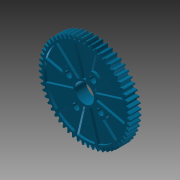
# Autodesk Inventor part: 12-0056_Gear
Saved by Autodesk Inventor 2015 SP1 (Build 190203100, 203)
## iProperties
Category: Gear Kit
Company: Autodesk Inc.
Created: 2014-11-29
Part Number: 12-0056_Gear
Material: Polystyrene, High Impact
Document SubType Name: Modeling
Designer: Matrix
Density: 1.022 g/cm^3
Appearance: Sky Blue Dark
Catalog Web Link: http://matrixrobotics.com/
Vendor: Matrix
Author: Autodesk Inc.
Autodesk Inventor part; units mm, degrees
ref_plane "YZ Plane" through (0, 0, 0) normal (1, 0, 0) x (0, 1, 0)
ref_plane "XZ Plane" through (0, 0, 0) normal (0, 1, 0) x (-1, 0, 0)
sketch "Sketch1" plane through (0, 0, 0) normal (0, 1, 0) x (-1, 0, 0)
  arc A0 (6.7425, 25.8863) -> (6.1348, 26.037) centre (0, 0) ccw
  arc A1 (5.9812, 26.2168) -> (6.1348, 26.037) centre (6.1806, 26.2317) ccw
  line L0 (5.9812, 26.2168) -> (5.8978, 27.33)
  line L1 (5.8978, 27.33) -> (5.7599, 28.1729)
  arc A2 (5.7599, 28.1729) -> (5.5196, 28.4193) centre (5.4639, 28.1245) ccw
  line L2 (5.5196, 28.4193) -> (5.2446, 28.4713)
  arc A3 (5.2446, 28.4713) -> (4.931, 28.3298) centre (5.1889, 28.1765) ccw
  line L3 (4.931, 28.3298) -> (4.4947, 27.5955)
  line L4 (4.4947, 27.5955) -> (4.0103, 26.5897)
  arc A4 (3.8017, 26.4785) -> (4.0103, 26.5897) centre (3.8301, 26.6764) ccw
  arc A5 (3.8017, 26.4785) -> (3.181, 26.5602) centre (0, 0) ccw
  arc A6 (3.0082, 26.7216) -> (3.181, 26.5602) centre (3.2047, 26.7588) ccw
  line L5 (3.0082, 26.7216) -> (2.8007, 27.8185)
  line L6 (2.8007, 27.8185) -> (2.5694, 28.6407)
  arc A7 (2.5694, 28.6407) -> (2.303, 28.8586) centre (2.2806, 28.5594) ccw
  line L7 (2.303, 28.8586) -> (2.0239, 28.8795)
  arc A8 (2.0239, 28.8795) -> (1.728, 28.7037) centre (2.0015, 28.5803) ccw
  line L8 (1.728, 28.7037) -> (1.3767, 27.9252)
  line L9 (1.3767, 27.9252) -> (1.008, 26.8715)
  arc A9 (0.8132, 26.7376) -> (1.008, 26.8715) centre (0.8192, 26.9375) ccw
  arc A10 (0.8132, 26.7376) -> (0.1872, 26.7493) centre (0, 0) ccw
  arc A11 (-0.0026, 26.8904) -> (0.1872, 26.7493) centre (0.1886, 26.9493) ccw
  line L10 (-0.0026, 26.8904) -> (-0.3316, 27.9572)
  line L11 (-0.3316, 27.9572) -> (-0.6535, 28.7483)
  arc A12 (-0.6535, 28.7483) -> (-0.9426, 28.935) centre (-0.9314, 28.6352) ccw
  line L12 (-0.9426, 28.935) -> (-1.2223, 28.9245)
  arc A13 (-1.2223, 28.9245) -> (-1.4966, 28.7167) centre (-1.2111, 28.6247) ccw
  line L13 (-1.7586, 27.9038) -> (-1.4966, 28.7167)
  line L14 (-1.7586, 27.9038) -> (-2.007, 26.8154)
  arc A14 (-2.1856, 26.6606) -> (-2.007, 26.8154) centre (-2.202, 26.8599) ccw
  arc A15 (-2.1856, 26.6606) -> (-2.809, 26.6021) centre (0, 0) ccw
  arc A16 (-3.0133, 26.721) -> (-2.809, 26.6021) centre (-2.83, 26.801) ccw
  line L15 (-3.0133, 26.721) -> (-3.4597, 27.7442)
  line L16 (-3.4597, 27.7442) -> (-3.8682, 28.4943)
  arc A17 (-3.8682, 28.4943) -> (-4.1764, 28.6475) centre (-4.1317, 28.3509) ccw
  line L17 (-4.1764, 28.6475) -> (-4.4531, 28.6058)
  arc A18 (-4.4531, 28.6058) -> (-4.7025, 28.3686) centre (-4.4084, 28.3091) ccw
  line L18 (-4.7025, 28.3686) -> (-4.8717, 27.5314)
  line L19 (-4.8717, 27.5314) -> (-4.9967, 26.4221)
  arc A19 (-5.1569, 26.2482) -> (-4.9967, 26.4221) centre (-5.1955, 26.4445) ccw
  arc A20 (-5.1569, 26.2482) -> (-5.7698, 26.1203) centre (0, 0) ccw
  arc A21 (-5.9862, 26.2156) -> (-5.7698, 26.1203) centre (-5.813, 26.3156) ccw
  line L20 (-5.9862, 26.2156) -> (-6.5444, 27.1824)
  line L21 (-6.5444, 27.1824) -> (-7.0343, 27.8821)
  arc A22 (-7.0343, 27.8821) -> (-7.3576, 27.9998) centre (-7.28, 27.71) ccw
  line L22 (-7.3576, 27.9998) -> (-7.628, 27.9273)
  arc A23 (-7.628, 27.9273) -> (-7.8492, 27.6637) centre (-7.5503, 27.6376) ccw
  line L23 (-7.8492, 27.6637) -> (-7.9236, 26.8128)
  line L24 (-7.9236, 26.8128) -> (-7.9236, 25.6965)
  arc A24 (-8.0633, 25.5058) -> (-7.9236, 25.6965) centre (-8.1236, 25.6965) ccw
  arc A25 (-8.0633, 25.5058) -> (-8.6581, 25.3101) centre (0, 0) ccw
  arc A26 (-8.8837, 25.3805) -> (-8.6581, 25.3101) centre (-8.7228, 25.4993) ccw
  line L25 (-8.8837, 25.3805) -> (-9.5467, 26.2788)
  line L26 (-9.5467, 26.2788) -> (-10.1118, 26.9192)
  arc A27 (-10.1118, 26.9192) -> (-10.4464, 26.9999) centre (-10.3368, 26.7207) ccw
  line L27 (-10.4464, 26.9999) -> (-10.7069, 26.8977)
  arc A28 (-10.7069, 26.8977) -> (-10.8972, 26.6109) centre (-10.5973, 26.6184) ccw
  line L28 (-10.8972, 26.6109) -> (-10.8759, 25.7571)
  line L29 (-10.8759, 25.7571) -> (-10.7509, 24.6477)
  arc A29 (-10.8684, 24.4426) -> (-10.7509, 24.6477) centre (-10.9496, 24.6253) ccw
  arc A30 (-10.8684, 24.4426) -> (-11.4375, 24.1815) centre (0, 0) ccw
  arc A31 (-11.6696, 24.2263) -> (-11.4375, 24.1815) centre (-11.523, 24.3623) ccw
  line L30 (-11.6696, 24.2263) -> (-12.4289, 25.0446)
  line L31 (-12.4289, 25.0446) -> (-13.0622, 25.6177)
  arc A32 (-13.0622, 25.6177) -> (-13.4037, 25.6605) centre (-13.2635, 25.3953) ccw
  line L32 (-13.4037, 25.6605) -> (-13.6511, 25.5298)
  arc A33 (-13.6511, 25.5298) -> (-13.8082, 25.2235) centre (-13.511, 25.2645) ccw
  line L33 (-13.8082, 25.2235) -> (-13.6914, 24.3774)
  line L34 (-13.6914, 24.3774) -> (-13.443, 23.289)
  arc A34 (-13.5368, 23.072) -> (-13.443, 23.289) centre (-13.638, 23.2445) ccw
  arc A35 (-13.5368, 23.072) -> (-14.073, 22.7489) centre (0, 0) ccw
  arc A36 (-14.3087, 22.7674) -> (-14.073, 22.7489) centre (-14.1783, 22.919) ccw
  line L35 (-14.3087, 22.7674) -> (-15.1549, 23.4956)
  line L36 (-15.1549, 23.4956) -> (-15.8484, 23.9942)
  arc A37 (-15.8484, 23.9942) -> (-16.1925, 23.9984) centre (-16.0235, 23.7506) ccw
  line L37 (-16.1925, 23.9984) -> (-16.4237, 23.8408)
  arc A38 (-16.4237, 23.8408) -> (-16.5455, 23.5189) centre (-16.2547, 23.5929) ccw
  line L38 (-16.5455, 23.5189) -> (-16.3347, 22.6912)
  line L39 (-16.3347, 22.6912) -> (-15.966, 21.6375)
  arc A39 (-16.0349, 21.4113) -> (-15.966, 21.6375) centre (-16.1548, 21.5714) ccw
  arc A40 (-16.0349, 21.4113) -> (-16.5316, 21.0302) centre (0, 0) ccw
  arc A41 (-16.7679, 21.0222) -> (-16.5316, 21.0302) centre (-16.6552, 21.1874) ccw
  line L40 (-16.7679, 21.0222) -> (-17.6903, 21.651)
  line L41 (-17.6903, 21.651) -> (-18.4352, 22.0688)
  arc A42 (-18.4352, 22.0688) -> (-18.7777, 22.0346) centre (-18.582, 21.8072) ccw
  line L42 (-18.7777, 22.0346) -> (-18.9898, 21.852)
  arc A43 (-18.9898, 21.852) -> (-19.0747, 21.5185) centre (-18.7941, 21.6246) ccw
  line L43 (-19.0747, 21.5185) -> (-18.7726, 20.7196)
  line L44 (-18.7726, 20.7196) -> (-18.2882, 19.7138)
  arc A44 (-18.3314, 19.4814) -> (-18.2882, 19.7138) centre (-18.4684, 19.627) ccw
  arc A45 (-18.3314, 19.4814) -> (-18.7823, 19.047) centre (0, 0) ccw
  arc A46 (-19.0162, 19.0126) -> (-18.7823, 19.047) centre (-18.9227, 19.1894) ccw
  line L45 (-19.0162, 19.0126) -> (-20.0032, 19.5342)
  line L46 (-20.0032, 19.5342) -> (-20.7902, 19.866)
  arc A47 (-20.7902, 19.866) -> (-21.1267, 19.7936) centre (-20.9068, 19.5895) ccw
  line L47 (-21.1267, 19.7936) -> (-21.317, 19.5884)
  arc A48 (-21.317, 19.5884) -> (-21.3641, 19.2475) centre (-21.0971, 19.3844) ccw
  line L48 (-21.3641, 19.2475) -> (-20.9744, 18.4875)
  line L49 (-20.9744, 18.4875) -> (-20.3805, 17.5422)
  arc A49 (-20.3973, 17.3064) -> (-20.3805, 17.5422) centre (-20.5498, 17.4358) ccw
  arc A50 (-20.3973, 17.3064) -> (-20.7968, 16.8243) centre (0, 0) ccw
  arc A51 (-21.0253, 16.7639) -> (-20.7968, 16.8243) centre (-20.9523, 16.9501) ccw
  line L50 (-21.0253, 16.7639) -> (-22.0645, 17.1717)
  line L51 (-22.8838, 17.4133) -> (-22.0645, 17.1717)
  arc A52 (-22.8838, 17.4133) -> (-23.21, 17.3037) centre (-22.9686, 17.1255) ccw
  line L52 (-23.21, 17.3037) -> (-23.3762, 17.0785)
  arc A53 (-23.3762, 17.0785) -> (-23.3848, 16.7345) centre (-23.1348, 16.9004) ccw
  line L53 (-23.3848, 16.7345) -> (-22.9125, 16.0228)
  line L54 (-22.9125, 16.0228) -> (-22.2164, 15.15)
  arc A54 (-22.2068, 14.9138) -> (-22.2164, 15.15) centre (-22.3728, 15.0253) ccw
  arc A55 (-22.2068, 14.9138) -> (-22.5497, 14.39) centre (0, 0) ccw
  arc A56 (-22.7701, 14.3044) -> (-22.5497, 14.39) centre (-22.7183, 14.4976) ccw
  line L55 (-22.7701, 14.3044) -> (-23.8484, 14.5933)
  line L56 (-23.8484, 14.5933) -> (-24.6896, 14.7416)
  arc A57 (-24.6896, 14.7416) -> (-25.0015, 14.5962) centre (-24.7417, 14.4462) ccw
  line L57 (-25.0015, 14.5962) -> (-25.1414, 14.3538)
  arc A58 (-25.1414, 14.3538) -> (-25.1114, 14.011) centre (-24.8816, 14.2038) ccw
  line L58 (-25.1114, 14.011) -> (-24.5624, 13.3567)
  line L59 (-24.5624, 13.3567) -> (-23.773, 12.5673)
  arc A59 (-23.737, 12.3337) -> (-23.773, 12.5673) centre (-23.9144, 12.4259) ccw
  arc A60 (-23.737, 12.3337) -> (-24.0191, 11.7747) centre (0, 0) ccw
  arc A61 (-24.2285, 11.665) -> (-24.0191, 11.7747) centre (-24.1987, 11.8628) ccw
  line L60 (-24.2285, 11.665) -> (-25.3324, 11.8314)
  line L61 (-25.3324, 11.8314) -> (-26.1849, 11.8846)
  arc A62 (-26.1849, 11.8846) -> (-26.4785, 11.7051) centre (-26.2035, 11.5852) ccw
  line L62 (-26.4785, 11.7051) -> (-26.5904, 11.4486)
  arc A63 (-26.5904, 11.4486) -> (-26.5222, 11.1113) centre (-26.3155, 11.3286) ccw
  line L63 (-26.5222, 11.1113) -> (-25.9034, 10.5226)
  line L64 (-25.9034, 10.5226) -> (-25.0306, 9.8265)
  arc A64 (-24.9686, 9.5984) -> (-25.0306, 9.8265) centre (-25.1553, 9.6702) ccw
  arc A65 (-24.9686, 9.5984) -> (-25.1864, 9.0114) centre (0, 0) ccw
  arc A66 (-25.3822, 8.8789) -> (-25.1864, 9.0114) centre (-25.3748, 9.0788) ccw
  line L65 (-25.3822, 8.8789) -> (-26.4978, 8.9207)
  line L66 (-26.4978, 8.9207) -> (-27.3509, 8.8781)
  arc A67 (-27.3509, 8.8781) -> (-27.6226, 8.6669) centre (-27.3359, 8.5785) ccw
  line L67 (-27.7051, 8.3994) -> (-27.6226, 8.6669)
  arc A68 (-27.7051, 8.3994) -> (-27.5995, 8.0719) centre (-27.4184, 8.311) ccw
  line L68 (-27.5995, 8.0719) -> (-26.9187, 7.5562)
  line L69 (-26.9187, 7.5562) -> (-25.9735, 6.9622)
  arc A69 (-25.8863, 6.7425) -> (-25.9735, 6.9622) centre (-26.0799, 6.7929) ccw
  arc A70 (-25.8863, 6.7425) -> (-26.037, 6.1348) centre (0, 0) ccw
  arc A71 (-26.2168, 5.9812) -> (-26.037, 6.1348) centre (-26.2317, 6.1806) ccw
  line L70 (-26.2168, 5.9812) -> (-27.33, 5.8978)
  line L71 (-27.33, 5.8978) -> (-28.1729, 5.7599)
  arc A72 (-28.1729, 5.7599) -> (-28.4193, 5.5196) centre (-28.1245, 5.4639) ccw
  line L72 (-28.4193, 5.5196) -> (-28.4713, 5.2446)
  arc A73 (-28.4713, 5.2446) -> (-28.3298, 4.931) centre (-28.1765, 5.1889) ccw
  line L73 (-28.3298, 4.931) -> (-27.5955, 4.4947)
  line L74 (-27.5955, 4.4947) -> (-26.5897, 4.0103)
  arc A74 (-26.4785, 3.8017) -> (-26.5897, 4.0103) centre (-26.6764, 3.8301) ccw
  arc A75 (-26.4785, 3.8017) -> (-26.5602, 3.181) centre (0, 0) ccw
  arc A76 (-26.7216, 3.0082) -> (-26.5602, 3.181) centre (-26.7588, 3.2047) ccw
  line L75 (-26.7216, 3.0082) -> (-27.8185, 2.8007)
  line L76 (-27.8185, 2.8007) -> (-28.6407, 2.5694)
  arc A77 (-28.6407, 2.5694) -> (-28.8586, 2.303) centre (-28.5594, 2.2806) ccw
  line L77 (-28.8586, 2.303) -> (-28.8795, 2.0239)
  arc A78 (-28.8795, 2.0239) -> (-28.7037, 1.728) centre (-28.5803, 2.0015) ccw
  line L78 (-28.7037, 1.728) -> (-27.9252, 1.3767)
  line L79 (-27.9252, 1.3767) -> (-26.8715, 1.008)
  arc A79 (-26.7376, 0.8132) -> (-26.8715, 1.008) centre (-26.9375, 0.8192) ccw
  arc A80 (-26.7376, 0.8132) -> (-26.7493, 0.1872) centre (0, 0) ccw
  arc A81 (-26.8904, -0.0026) -> (-26.7493, 0.1872) centre (-26.9493, 0.1886) ccw
  line L80 (-26.8904, -0.0026) -> (-27.9572, -0.3316)
  line L81 (-27.9572, -0.3316) -> (-28.7483, -0.6535)
  arc A82 (-28.7483, -0.6535) -> (-28.935, -0.9426) centre (-28.6352, -0.9314) ccw
  line L82 (-28.935, -0.9426) -> (-28.9245, -1.2223)
  arc A83 (-28.9245, -1.2223) -> (-28.7167, -1.4966) centre (-28.6247, -1.2111) ccw
  line L83 (-27.9038, -1.7586) -> (-28.7167, -1.4966)
  line L84 (-27.9038, -1.7586) -> (-26.8154, -2.007)
  arc A84 (-26.6606, -2.1856) -> (-26.8154, -2.007) centre (-26.8599, -2.202) ccw
  arc A85 (-26.6606, -2.1856) -> (-26.6021, -2.809) centre (0, 0) ccw
  arc A86 (-26.721, -3.0133) -> (-26.6021, -2.809) centre (-26.801, -2.83) ccw
  line L85 (-26.721, -3.0133) -> (-27.7442, -3.4597)
  line L86 (-27.7442, -3.4597) -> (-28.4943, -3.8682)
  arc A87 (-28.4943, -3.8682) -> (-28.6475, -4.1764) centre (-28.3509, -4.1317) ccw
  line L87 (-28.6475, -4.1764) -> (-28.6058, -4.4531)
  arc A88 (-28.6058, -4.4531) -> (-28.3686, -4.7025) centre (-28.3091, -4.4084) ccw
  line L88 (-28.3686, -4.7025) -> (-27.5314, -4.8717)
  line L89 (-27.5314, -4.8717) -> (-26.4221, -4.9967)
  arc A89 (-26.2482, -5.1569) -> (-26.4221, -4.9967) centre (-26.4445, -5.1955) ccw
  arc A90 (-26.2482, -5.1569) -> (-26.1203, -5.7698) centre (0, 0) ccw
  arc A91 (-26.2156, -5.9862) -> (-26.1203, -5.7698) centre (-26.3156, -5.813) ccw
  line L90 (-26.2156, -5.9862) -> (-27.1824, -6.5444)
  line L91 (-27.1824, -6.5444) -> (-27.8821, -7.0343)
  arc A92 (-27.8821, -7.0343) -> (-27.9998, -7.3576) centre (-27.71, -7.28) ccw
  line L92 (-27.9998, -7.3576) -> (-27.9273, -7.628)
  arc A93 (-27.9273, -7.628) -> (-27.6637, -7.8492) centre (-27.6376, -7.5503) ccw
  line L93 (-27.6637, -7.8492) -> (-26.8128, -7.9236)
  line L94 (-26.8128, -7.9236) -> (-25.6965, -7.9236)
  arc A94 (-25.5058, -8.0633) -> (-25.6965, -7.9236) centre (-25.6965, -8.1236) ccw
  arc A95 (-25.5058, -8.0633) -> (-25.3101, -8.6581) centre (0, 0) ccw
  arc A96 (-25.3805, -8.8837) -> (-25.3101, -8.6581) centre (-25.4993, -8.7228) ccw
  line L95 (-25.3805, -8.8837) -> (-26.2788, -9.5467)
  line L96 (-26.2788, -9.5467) -> (-26.9192, -10.1118)
  arc A97 (-26.9192, -10.1118) -> (-26.9999, -10.4464) centre (-26.7207, -10.3368) ccw
  line L97 (-26.9999, -10.4464) -> (-26.8977, -10.7069)
  arc A98 (-26.8977, -10.7069) -> (-26.6109, -10.8972) centre (-26.6184, -10.5973) ccw
  line L98 (-26.6109, -10.8972) -> (-25.7571, -10.8759)
  line L99 (-25.7571, -10.8759) -> (-24.6477, -10.7509)
  arc A99 (-24.4426, -10.8684) -> (-24.6477, -10.7509) centre (-24.6253, -10.9496) ccw
  arc A100 (-24.4426, -10.8684) -> (-24.1815, -11.4375) centre (0, 0) ccw
  arc A101 (-24.2263, -11.6696) -> (-24.1815, -11.4375) centre (-24.3623, -11.523) ccw
  line L100 (-24.2263, -11.6696) -> (-25.0446, -12.4289)
  line L101 (-25.0446, -12.4289) -> (-25.6177, -13.0622)
  arc A102 (-25.6177, -13.0622) -> (-25.6605, -13.4037) centre (-25.3953, -13.2635) ccw
  line L102 (-25.6605, -13.4037) -> (-25.5298, -13.6511)
  arc A103 (-25.5298, -13.6511) -> (-25.2235, -13.8082) centre (-25.2645, -13.511) ccw
  line L103 (-25.2235, -13.8082) -> (-24.3774, -13.6914)
  line L104 (-24.3774, -13.6914) -> (-23.289, -13.443)
  arc A104 (-23.072, -13.5368) -> (-23.289, -13.443) centre (-23.2445, -13.638) ccw
  arc A105 (-23.072, -13.5368) -> (-22.7489, -14.073) centre (0, 0) ccw
  arc A106 (-22.7674, -14.3087) -> (-22.7489, -14.073) centre (-22.919, -14.1783) ccw
  line L105 (-22.7674, -14.3087) -> (-23.4956, -15.1549)
  line L106 (-23.4956, -15.1549) -> (-23.9942, -15.8484)
  arc A107 (-23.9942, -15.8484) -> (-23.9984, -16.1925) centre (-23.7506, -16.0235) ccw
  line L107 (-23.9984, -16.1925) -> (-23.8408, -16.4237)
  arc A108 (-23.8408, -16.4237) -> (-23.5189, -16.5455) centre (-23.5929, -16.2547) ccw
  line L108 (-23.5189, -16.5455) -> (-22.6912, -16.3347)
  line L109 (-22.6912, -16.3347) -> (-21.6375, -15.966)
  arc A109 (-21.4113, -16.0349) -> (-21.6375, -15.966) centre (-21.5714, -16.1548) ccw
  arc A110 (-21.4113, -16.0349) -> (-21.0302, -16.5316) centre (0, 0) ccw
  arc A111 (-21.0222, -16.7679) -> (-21.0302, -16.5316) centre (-21.1874, -16.6552) ccw
  line L110 (-21.0222, -16.7679) -> (-21.651, -17.6903)
  line L111 (-21.651, -17.6903) -> (-22.0688, -18.4352)
  arc A112 (-22.0688, -18.4352) -> (-22.0346, -18.7777) centre (-21.8072, -18.582) ccw
  line L112 (-22.0346, -18.7777) -> (-21.852, -18.9898)
  arc A113 (-21.852, -18.9898) -> (-21.5185, -19.0747) centre (-21.6246, -18.7941) ccw
  line L113 (-21.5185, -19.0747) -> (-20.7196, -18.7726)
  line L114 (-20.7196, -18.7726) -> (-19.7138, -18.2882)
  arc A114 (-19.4814, -18.3314) -> (-19.7138, -18.2882) centre (-19.627, -18.4684) ccw
  arc A115 (-19.4814, -18.3314) -> (-19.047, -18.7823) centre (0, 0) ccw
  arc A116 (-19.0126, -19.0162) -> (-19.047, -18.7823) centre (-19.1894, -18.9227) ccw
  line L115 (-19.0126, -19.0162) -> (-19.5342, -20.0032)
  line L116 (-19.5342, -20.0032) -> (-19.866, -20.7902)
  arc A117 (-19.866, -20.7902) -> (-19.7936, -21.1267) centre (-19.5895, -20.9068) ccw
  line L117 (-19.7936, -21.1267) -> (-19.5884, -21.317)
  arc A118 (-19.5884, -21.317) -> (-19.2475, -21.3641) centre (-19.3844, -21.0971) ccw
  line L118 (-19.2475, -21.3641) -> (-18.4875, -20.9744)
  line L119 (-18.4875, -20.9744) -> (-17.5422, -20.3805)
  arc A119 (-17.3064, -20.3973) -> (-17.5422, -20.3805) centre (-17.4358, -20.5498) ccw
  arc A120 (-17.3064, -20.3973) -> (-16.8243, -20.7968) centre (0, 0) ccw
  arc A121 (-16.7639, -21.0253) -> (-16.8243, -20.7968) centre (-16.9501, -20.9523) ccw
  line L120 (-16.7639, -21.0253) -> (-17.1717, -22.0645)
  line L121 (-17.4133, -22.8838) -> (-17.1717, -22.0645)
  arc A122 (-17.4133, -22.8838) -> (-17.3037, -23.21) centre (-17.1255, -22.9686) ccw
  line L122 (-17.3037, -23.21) -> (-17.0785, -23.3762)
  arc A123 (-17.0785, -23.3762) -> (-16.7345, -23.3848) centre (-16.9004, -23.1348) ccw
  line L123 (-16.7345, -23.3848) -> (-16.0228, -22.9125)
  line L124 (-16.0228, -22.9125) -> (-15.15, -22.2164)
  arc A124 (-14.9138, -22.2068) -> (-15.15, -22.2164) centre (-15.0253, -22.3728) ccw
  arc A125 (-14.9138, -22.2068) -> (-14.39, -22.5497) centre (0, 0) ccw
  arc A126 (-14.3044, -22.7701) -> (-14.39, -22.5497) centre (-14.4976, -22.7183) ccw
  line L125 (-14.3044, -22.7701) -> (-14.5933, -23.8484)
  line L126 (-14.5933, -23.8484) -> (-14.7416, -24.6896)
  arc A127 (-14.7416, -24.6896) -> (-14.5962, -25.0015) centre (-14.4462, -24.7417) ccw
  line L127 (-14.5962, -25.0015) -> (-14.3538, -25.1414)
  arc A128 (-14.3538, -25.1414) -> (-14.011, -25.1114) centre (-14.2038, -24.8816) ccw
  line L128 (-14.011, -25.1114) -> (-13.3567, -24.5624)
  line L129 (-13.3567, -24.5624) -> (-12.5673, -23.773)
  arc A129 (-12.3337, -23.737) -> (-12.5673, -23.773) centre (-12.4259, -23.9144) ccw
  arc A130 (-12.3337, -23.737) -> (-11.7747, -24.0191) centre (0, 0) ccw
  arc A131 (-11.665, -24.2285) -> (-11.7747, -24.0191) centre (-11.8628, -24.1987) ccw
  line L130 (-11.665, -24.2285) -> (-11.8314, -25.3324)
  line L131 (-11.8314, -25.3324) -> (-11.8846, -26.1849)
  arc A132 (-11.8846, -26.1849) -> (-11.7051, -26.4785) centre (-11.5852, -26.2035) ccw
  line L132 (-11.7051, -26.4785) -> (-11.4486, -26.5904)
  arc A133 (-11.4486, -26.5904) -> (-11.1113, -26.5222) centre (-11.3286, -26.3155) ccw
  line L133 (-11.1113, -26.5222) -> (-10.5226, -25.9034)
  line L134 (-10.5226, -25.9034) -> (-9.8265, -25.0306)
  arc A134 (-9.5984, -24.9686) -> (-9.8265, -25.0306) centre (-9.6702, -25.1553) ccw
  arc A135 (-9.5984, -24.9686) -> (-9.0114, -25.1864) centre (0, 0) ccw
  arc A136 (-8.8789, -25.3822) -> (-9.0114, -25.1864) centre (-9.0788, -25.3748) ccw
  line L135 (-8.8789, -25.3822) -> (-8.9207, -26.4978)
  line L136 (-8.9207, -26.4978) -> (-8.8781, -27.3509)
  arc A137 (-8.8781, -27.3509) -> (-8.6669, -27.6226) centre (-8.5785, -27.3359) ccw
  line L137 (-8.3994, -27.7051) -> (-8.6669, -27.6226)
  arc A138 (-8.3994, -27.7051) -> (-8.0719, -27.5995) centre (-8.311, -27.4184) ccw
  line L138 (-8.0719, -27.5995) -> (-7.5562, -26.9187)
  line L139 (-7.5562, -26.9187) -> (-6.9622, -25.9735)
  arc A139 (-6.7425, -25.8863) -> (-6.9622, -25.9735) centre (-6.7929, -26.0799) ccw
  arc A140 (-6.7425, -25.8863) -> (-6.1348, -26.037) centre (0, 0) ccw
  arc A141 (-5.9812, -26.2168) -> (-6.1348, -26.037) centre (-6.1806, -26.2317) ccw
  line L140 (-5.9812, -26.2168) -> (-5.8978, -27.33)
  line L141 (-5.8978, -27.33) -> (-5.7599, -28.1729)
  arc A142 (-5.7599, -28.1729) -> (-5.5196, -28.4193) centre (-5.4639, -28.1245) ccw
  line L142 (-5.5196, -28.4193) -> (-5.2446, -28.4713)
  arc A143 (-5.2446, -28.4713) -> (-4.931, -28.3298) centre (-5.1889, -28.1765) ccw
  line L143 (-4.931, -28.3298) -> (-4.4947, -27.5955)
  line L144 (-4.4947, -27.5955) -> (-4.0103, -26.5897)
  arc A144 (-3.8017, -26.4785) -> (-4.0103, -26.5897) centre (-3.8301, -26.6764) ccw
  arc A145 (-3.8017, -26.4785) -> (-3.181, -26.5602) centre (0, 0) ccw
  arc A146 (-3.0082, -26.7216) -> (-3.181, -26.5602) centre (-3.2047, -26.7588) ccw
  line L145 (-3.0082, -26.7216) -> (-2.8007, -27.8185)
  line L146 (-2.8007, -27.8185) -> (-2.5694, -28.6407)
  arc A147 (-2.5694, -28.6407) -> (-2.303, -28.8586) centre (-2.2806, -28.5594) ccw
  line L147 (-2.303, -28.8586) -> (-2.0239, -28.8795)
  arc A148 (-2.0239, -28.8795) -> (-1.728, -28.7037) centre (-2.0015, -28.5803) ccw
  line L148 (-1.728, -28.7037) -> (-1.3767, -27.9252)
  line L149 (-1.3767, -27.9252) -> (-1.008, -26.8715)
  arc A149 (-0.8132, -26.7376) -> (-1.008, -26.8715) centre (-0.8192, -26.9375) ccw
  arc A150 (-0.8132, -26.7376) -> (-0.1872, -26.7493) centre (0, 0) ccw
  arc A151 (0.0026, -26.8904) -> (-0.1872, -26.7493) centre (-0.1886, -26.9493) ccw
  line L150 (0.0026, -26.8904) -> (0.3316, -27.9572)
  line L151 (0.3316, -27.9572) -> (0.6535, -28.7483)
  arc A152 (0.6535, -28.7483) -> (0.9426, -28.935) centre (0.9314, -28.6352) ccw
  line L152 (0.9426, -28.935) -> (1.2223, -28.9245)
  arc A153 (1.2223, -28.9245) -> (1.4966, -28.7167) centre (1.2111, -28.6247) ccw
  line L153 (1.7586, -27.9038) -> (1.4966, -28.7167)
  line L154 (1.7586, -27.9038) -> (2.007, -26.8154)
  arc A154 (2.1856, -26.6606) -> (2.007, -26.8154) centre (2.202, -26.8599) ccw
  arc A155 (2.1856, -26.6606) -> (2.809, -26.6021) centre (0, 0) ccw
  arc A156 (3.0133, -26.721) -> (2.809, -26.6021) centre (2.83, -26.801) ccw
  line L155 (3.0133, -26.721) -> (3.4597, -27.7442)
  line L156 (3.4597, -27.7442) -> (3.8682, -28.4943)
  arc A157 (3.8682, -28.4943) -> (4.1764, -28.6475) centre (4.1317, -28.3509) ccw
  line L157 (4.1764, -28.6475) -> (4.4531, -28.6058)
  arc A158 (4.4531, -28.6058) -> (4.7025, -28.3686) centre (4.4084, -28.3091) ccw
  line L158 (4.7025, -28.3686) -> (4.8717, -27.5314)
  line L159 (4.8717, -27.5314) -> (4.9967, -26.4221)
  arc A159 (5.1569, -26.2482) -> (4.9967, -26.4221) centre (5.1955, -26.4445) ccw
  arc A160 (5.1569, -26.2482) -> (5.7698, -26.1203) centre (0, 0) ccw
  arc A161 (5.9862, -26.2156) -> (5.7698, -26.1203) centre (5.813, -26.3156) ccw
  line L160 (5.9862, -26.2156) -> (6.5444, -27.1824)
  line L161 (6.5444, -27.1824) -> (7.0343, -27.8821)
  arc A162 (7.0343, -27.8821) -> (7.3576, -27.9998) centre (7.28, -27.71) ccw
  line L162 (7.3576, -27.9998) -> (7.628, -27.9273)
  arc A163 (7.628, -27.9273) -> (7.8492, -27.6637) centre (7.5503, -27.6376) ccw
  line L163 (7.8492, -27.6637) -> (7.9236, -26.8128)
  line L164 (7.9236, -26.8128) -> (7.9236, -25.6965)
  arc A164 (8.0633, -25.5058) -> (7.9236, -25.6965) centre (8.1236, -25.6965) ccw
  arc A165 (8.0633, -25.5058) -> (8.6581, -25.3101) centre (0, 0) ccw
  arc A166 (8.8837, -25.3805) -> (8.6581, -25.3101) centre (8.7228, -25.4993) ccw
  line L165 (8.8837, -25.3805) -> (9.5467, -26.2788)
  line L166 (9.5467, -26.2788) -> (10.1118, -26.9192)
  arc A167 (10.1118, -26.9192) -> (10.4464, -26.9999) centre (10.3368, -26.7207) ccw
  line L167 (10.4464, -26.9999) -> (10.7069, -26.8977)
  arc A168 (10.7069, -26.8977) -> (10.8972, -26.6109) centre (10.5973, -26.6184) ccw
  line L168 (10.8972, -26.6109) -> (10.8759, -25.7571)
  line L169 (10.8759, -25.7571) -> (10.7509, -24.6477)
  arc A169 (10.8684, -24.4426) -> (10.7509, -24.6477) centre (10.9496, -24.6253) ccw
  arc A170 (10.8684, -24.4426) -> (11.4375, -24.1815) centre (0, 0) ccw
  arc A171 (11.6696, -24.2263) -> (11.4375, -24.1815) centre (11.523, -24.3623) ccw
  line L170 (11.6696, -24.2263) -> (12.4289, -25.0446)
  line L171 (12.4289, -25.0446) -> (13.0622, -25.6177)
  arc A172 (13.0622, -25.6177) -> (13.4037, -25.6605) centre (13.2635, -25.3953) ccw
  line L172 (13.4037, -25.6605) -> (13.6511, -25.5298)
  arc A173 (13.6511, -25.5298) -> (13.8082, -25.2235) centre (13.511, -25.2645) ccw
  line L173 (13.8082, -25.2235) -> (13.6914, -24.3774)
  line L174 (13.6914, -24.3774) -> (13.443, -23.289)
  arc A174 (13.5368, -23.072) -> (13.443, -23.289) centre (13.638, -23.2445) ccw
  arc A175 (13.5368, -23.072) -> (14.073, -22.7489) centre (0, 0) ccw
  arc A176 (14.3087, -22.7674) -> (14.073, -22.7489) centre (14.1783, -22.919) ccw
  line L175 (14.3087, -22.7674) -> (15.1549, -23.4956)
  line L176 (15.1549, -23.4956) -> (15.8484, -23.9942)
  arc A177 (15.8484, -23.9942) -> (16.1925, -23.9984) centre (16.0235, -23.7506) ccw
  line L177 (16.1925, -23.9984) -> (16.4237, -23.8408)
  arc A178 (16.4237, -23.8408) -> (16.5455, -23.5189) centre (16.2547, -23.5929) ccw
  line L178 (16.5455, -23.5189) -> (16.3347, -22.6912)
  line L179 (16.3347, -22.6912) -> (15.966, -21.6375)
  arc A179 (16.0349, -21.4113) -> (15.966, -21.6375) centre (16.1548, -21.5714) ccw
  arc A180 (16.0349, -21.4113) -> (16.5316, -21.0302) centre (0, 0) ccw
  arc A181 (16.7679, -21.0222) -> (16.5316, -21.0302) centre (16.6552, -21.1874) ccw
  line L180 (16.7679, -21.0222) -> (17.6903, -21.651)
  line L181 (17.6903, -21.651) -> (18.4352, -22.0688)
  arc A182 (18.4352, -22.0688) -> (18.7777, -22.0346) centre (18.582, -21.8072) ccw
  line L182 (18.7777, -22.0346) -> (18.9898, -21.852)
  arc A183 (18.9898, -21.852) -> (19.0747, -21.5185) centre (18.7941, -21.6246) ccw
  line L183 (19.0747, -21.5185) -> (18.7726, -20.7196)
  line L184 (18.7726, -20.7196) -> (18.2882, -19.7138)
  arc A184 (18.3314, -19.4814) -> (18.2882, -19.7138) centre (18.4684, -19.627) ccw
  arc A185 (18.3314, -19.4814) -> (18.7823, -19.047) centre (0, 0) ccw
  arc A186 (19.0162, -19.0126) -> (18.7823, -19.047) centre (18.9227, -19.1894) ccw
  line L185 (19.0162, -19.0126) -> (20.0032, -19.5342)
  line L186 (20.0032, -19.5342) -> (20.7902, -19.866)
  arc A187 (20.7902, -19.866) -> (21.1267, -19.7936) centre (20.9068, -19.5895) ccw
  line L187 (21.1267, -19.7936) -> (21.317, -19.5884)
  arc A188 (21.317, -19.5884) -> (21.3641, -19.2475) centre (21.0971, -19.3844) ccw
  line L188 (21.3641, -19.2475) -> (20.9744, -18.4875)
  line L189 (20.9744, -18.4875) -> (20.3805, -17.5422)
  arc A189 (20.3973, -17.3064) -> (20.3805, -17.5422) centre (20.5498, -17.4358) ccw
  arc A190 (20.3973, -17.3064) -> (20.7968, -16.8243) centre (0, 0) ccw
  arc A191 (21.0253, -16.7639) -> (20.7968, -16.8243) centre (20.9523, -16.9501) ccw
  line L190 (21.0253, -16.7639) -> (22.0645, -17.1717)
  line L191 (22.8838, -17.4133) -> (22.0645, -17.1717)
  arc A192 (22.8838, -17.4133) -> (23.21, -17.3037) centre (22.9686, -17.1255) ccw
  line L192 (23.21, -17.3037) -> (23.3762, -17.0785)
  arc A193 (23.3762, -17.0785) -> (23.3848, -16.7345) centre (23.1348, -16.9004) ccw
  line L193 (23.3848, -16.7345) -> (22.9125, -16.0228)
  line L194 (22.9125, -16.0228) -> (22.2164, -15.15)
  arc A194 (22.2068, -14.9138) -> (22.2164, -15.15) centre (22.3728, -15.0253) ccw
  arc A195 (22.2068, -14.9138) -> (22.5497, -14.39) centre (0, 0) ccw
  arc A196 (22.7701, -14.3044) -> (22.5497, -14.39) centre (22.7183, -14.4976) ccw
  line L195 (22.7701, -14.3044) -> (23.8484, -14.5933)
  line L196 (23.8484, -14.5933) -> (24.6896, -14.7416)
  arc A197 (24.6896, -14.7416) -> (25.0015, -14.5962) centre (24.7417, -14.4462) ccw
  line L197 (25.0015, -14.5962) -> (25.1414, -14.3538)
  arc A198 (25.1414, -14.3538) -> (25.1114, -14.011) centre (24.8816, -14.2038) ccw
  line L198 (25.1114, -14.011) -> (24.5624, -13.3567)
  line L199 (24.5624, -13.3567) -> (23.773, -12.5673)
  arc A199 (23.737, -12.3337) -> (23.773, -12.5673) centre (23.9144, -12.4259) ccw
  arc A200 (23.737, -12.3337) -> (24.0191, -11.7747) centre (0, 0) ccw
  arc A201 (24.2285, -11.665) -> (24.0191, -11.7747) centre (24.1987, -11.8628) ccw
  line L200 (24.2285, -11.665) -> (25.3324, -11.8314)
  line L201 (25.3324, -11.8314) -> (26.1849, -11.8846)
  arc A202 (26.1849, -11.8846) -> (26.4785, -11.7051) centre (26.2035, -11.5852) ccw
  line L202 (26.4785, -11.7051) -> (26.5904, -11.4486)
  arc A203 (26.5904, -11.4486) -> (26.5222, -11.1113) centre (26.3155, -11.3286) ccw
  line L203 (26.5222, -11.1113) -> (25.9034, -10.5226)
  line L204 (25.9034, -10.5226) -> (25.0306, -9.8265)
  arc A204 (24.9686, -9.5984) -> (25.0306, -9.8265) centre (25.1553, -9.6702) ccw
  arc A205 (24.9686, -9.5984) -> (25.1864, -9.0114) centre (0, 0) ccw
  arc A206 (25.3822, -8.8789) -> (25.1864, -9.0114) centre (25.3748, -9.0788) ccw
  line L205 (25.3822, -8.8789) -> (26.4978, -8.9207)
  line L206 (26.4978, -8.9207) -> (27.3509, -8.8781)
  arc A207 (27.3509, -8.8781) -> (27.6226, -8.6669) centre (27.3359, -8.5785) ccw
  line L207 (27.7051, -8.3994) -> (27.6226, -8.6669)
  arc A208 (27.7051, -8.3994) -> (27.5995, -8.0719) centre (27.4184, -8.311) ccw
  line L208 (27.5995, -8.0719) -> (26.9187, -7.5562)
  line L209 (26.9187, -7.5562) -> (25.9735, -6.9622)
  arc A209 (25.8863, -6.7425) -> (25.9735, -6.9622) centre (26.0799, -6.7929) ccw
  arc A210 (25.8863, -6.7425) -> (26.037, -6.1348) centre (0, 0) ccw
  arc A211 (26.2168, -5.9812) -> (26.037, -6.1348) centre (26.2317, -6.1806) ccw
  line L210 (26.2168, -5.9812) -> (27.33, -5.8978)
  line L211 (27.33, -5.8978) -> (28.1729, -5.7599)
  arc A212 (28.1729, -5.7599) -> (28.4193, -5.5196) centre (28.1245, -5.4639) ccw
  line L212 (28.4193, -5.5196) -> (28.4713, -5.2446)
  arc A213 (28.4713, -5.2446) -> (28.3298, -4.931) centre (28.1765, -5.1889) ccw
  line L213 (28.3298, -4.931) -> (27.5955, -4.4947)
  line L214 (27.5955, -4.4947) -> (26.5897, -4.0103)
  arc A214 (26.4785, -3.8017) -> (26.5897, -4.0103) centre (26.6764, -3.8301) ccw
  arc A215 (26.4785, -3.8017) -> (26.5602, -3.181) centre (0, 0) ccw
  arc A216 (26.7216, -3.0082) -> (26.5602, -3.181) centre (26.7588, -3.2047) ccw
  line L215 (26.7216, -3.0082) -> (27.8185, -2.8007)
  line L216 (27.8185, -2.8007) -> (28.6407, -2.5694)
  arc A217 (28.6407, -2.5694) -> (28.8586, -2.303) centre (28.5594, -2.2806) ccw
  line L217 (28.8586, -2.303) -> (28.8795, -2.0239)
  arc A218 (28.8795, -2.0239) -> (28.7037, -1.728) centre (28.5803, -2.0015) ccw
  line L218 (28.7037, -1.728) -> (27.9252, -1.3767)
  line L219 (27.9252, -1.3767) -> (26.8715, -1.008)
  arc A219 (26.7376, -0.8132) -> (26.8715, -1.008) centre (26.9375, -0.8192) ccw
  arc A220 (26.7376, -0.8132) -> (26.7493, -0.1872) centre (0, 0) ccw
  arc A221 (26.8904, 0.0026) -> (26.7493, -0.1872) centre (26.9493, -0.1886) ccw
  line L220 (26.8904, 0.0026) -> (27.9572, 0.3316)
  line L221 (27.9572, 0.3316) -> (28.7483, 0.6535)
  arc A222 (28.7483, 0.6535) -> (28.935, 0.9426) centre (28.6352, 0.9314) ccw
  line L222 (28.935, 0.9426) -> (28.9245, 1.2223)
  arc A223 (28.9245, 1.2223) -> (28.7167, 1.4966) centre (28.6247, 1.2111) ccw
  line L223 (27.9038, 1.7586) -> (28.7167, 1.4966)
  line L224 (27.9038, 1.7586) -> (26.8154, 2.007)
  arc A224 (26.6606, 2.1856) -> (26.8154, 2.007) centre (26.8599, 2.202) ccw
  arc A225 (26.6606, 2.1856) -> (26.6021, 2.809) centre (0, 0) ccw
  arc A226 (26.721, 3.0133) -> (26.6021, 2.809) centre (26.801, 2.83) ccw
  line L225 (26.721, 3.0133) -> (27.7442, 3.4597)
  line L226 (27.7442, 3.4597) -> (28.4943, 3.8682)
  arc A227 (28.4943, 3.8682) -> (28.6475, 4.1764) centre (28.3509, 4.1317) ccw
  line L227 (28.6475, 4.1764) -> (28.6058, 4.4531)
  arc A228 (28.6058, 4.4531) -> (28.3686, 4.7025) centre (28.3091, 4.4084) ccw
  line L228 (28.3686, 4.7025) -> (27.5314, 4.8717)
  line L229 (27.5314, 4.8717) -> (26.4221, 4.9967)
  arc A229 (26.2482, 5.1569) -> (26.4221, 4.9967) centre (26.4445, 5.1955) ccw
  arc A230 (26.2482, 5.1569) -> (26.1203, 5.7698) centre (0, 0) ccw
  arc A231 (26.2156, 5.9862) -> (26.1203, 5.7698) centre (26.3156, 5.813) ccw
  line L230 (26.2156, 5.9862) -> (27.1824, 6.5444)
  line L231 (27.1824, 6.5444) -> (27.8821, 7.0343)
  arc A232 (27.8821, 7.0343) -> (27.9998, 7.3576) centre (27.71, 7.28) ccw
  line L232 (27.9998, 7.3576) -> (27.9273, 7.628)
  arc A233 (27.9273, 7.628) -> (27.6637, 7.8492) centre (27.6376, 7.5503) ccw
  line L233 (27.6637, 7.8492) -> (26.8128, 7.9236)
  line L234 (26.8128, 7.9236) -> (25.6965, 7.9236)
  arc A234 (25.5058, 8.0633) -> (25.6965, 7.9236) centre (25.6965, 8.1236) ccw
  arc A235 (25.5058, 8.0633) -> (25.3101, 8.6581) centre (0, 0) ccw
  arc A236 (25.3805, 8.8837) -> (25.3101, 8.6581) centre (25.4993, 8.7228) ccw
  line L235 (25.3805, 8.8837) -> (26.2788, 9.5467)
  line L236 (26.2788, 9.5467) -> (26.9192, 10.1118)
  arc A237 (26.9192, 10.1118) -> (26.9999, 10.4464) centre (26.7207, 10.3368) ccw
  line L237 (26.9999, 10.4464) -> (26.8977, 10.7069)
  arc A238 (26.8977, 10.7069) -> (26.6109, 10.8972) centre (26.6184, 10.5973) ccw
  line L238 (26.6109, 10.8972) -> (25.7571, 10.8759)
  line L239 (25.7571, 10.8759) -> (24.6477, 10.7509)
  arc A239 (24.4426, 10.8684) -> (24.6477, 10.7509) centre (24.6253, 10.9496) ccw
  arc A240 (24.4426, 10.8684) -> (24.1815, 11.4375) centre (0, 0) ccw
  arc A241 (24.2263, 11.6696) -> (24.1815, 11.4375) centre (24.3623, 11.523) ccw
  line L240 (24.2263, 11.6696) -> (25.0446, 12.4289)
  line L241 (25.0446, 12.4289) -> (25.6177, 13.0622)
  arc A242 (25.6177, 13.0622) -> (25.6605, 13.4037) centre (25.3953, 13.2635) ccw
  line L242 (25.6605, 13.4037) -> (25.5298, 13.6511)
  arc A243 (25.5298, 13.6511) -> (25.2235, 13.8082) centre (25.2645, 13.511) ccw
  line L243 (25.2235, 13.8082) -> (24.3774, 13.6914)
  line L244 (24.3774, 13.6914) -> (23.289, 13.443)
  arc A244 (23.072, 13.5368) -> (23.289, 13.443) centre (23.2445, 13.638) ccw
  arc A245 (23.072, 13.5368) -> (22.7489, 14.073) centre (0, 0) ccw
  arc A246 (22.7674, 14.3087) -> (22.7489, 14.073) centre (22.919, 14.1783) ccw
  line L245 (22.7674, 14.3087) -> (23.4956, 15.1549)
  line L246 (23.4956, 15.1549) -> (23.9942, 15.8484)
  arc A247 (23.9942, 15.8484) -> (23.9984, 16.1925) centre (23.7506, 16.0235) ccw
  line L247 (23.9984, 16.1925) -> (23.8408, 16.4237)
  arc A248 (23.8408, 16.4237) -> (23.5189, 16.5455) centre (23.5929, 16.2547) ccw
  line L248 (23.5189, 16.5455) -> (22.6912, 16.3347)
  line L249 (22.6912, 16.3347) -> (21.6375, 15.966)
  arc A249 (21.4113, 16.0349) -> (21.6375, 15.966) centre (21.5714, 16.1548) ccw
  arc A250 (21.4113, 16.0349) -> (21.0302, 16.5316) centre (0, 0) ccw
  arc A251 (21.0222, 16.7679) -> (21.0302, 16.5316) centre (21.1874, 16.6552) ccw
  line L250 (21.0222, 16.7679) -> (21.651, 17.6903)
  line L251 (21.651, 17.6903) -> (22.0688, 18.4352)
  arc A252 (22.0688, 18.4352) -> (22.0346, 18.7777) centre (21.8072, 18.582) ccw
  line L252 (22.0346, 18.7777) -> (21.852, 18.9898)
  arc A253 (21.852, 18.9898) -> (21.5185, 19.0747) centre (21.6246, 18.7941) ccw
  line L253 (21.5185, 19.0747) -> (20.7196, 18.7726)
  line L254 (20.7196, 18.7726) -> (19.7138, 18.2882)
  arc A254 (19.4814, 18.3314) -> (19.7138, 18.2882) centre (19.627, 18.4684) ccw
  arc A255 (19.4814, 18.3314) -> (19.047, 18.7823) centre (0, 0) ccw
  arc A256 (19.0126, 19.0162) -> (19.047, 18.7823) centre (19.1894, 18.9227) ccw
  line L255 (19.0126, 19.0162) -> (19.5342, 20.0032)
  line L256 (19.5342, 20.0032) -> (19.866, 20.7902)
  arc A257 (19.866, 20.7902) -> (19.7936, 21.1267) centre (19.5895, 20.9068) ccw
  line L257 (19.7936, 21.1267) -> (19.5884, 21.317)
  arc A258 (19.5884, 21.317) -> (19.2475, 21.3641) centre (19.3844, 21.0971) ccw
  line L258 (19.2475, 21.3641) -> (18.4875, 20.9744)
  line L259 (18.4875, 20.9744) -> (17.5422, 20.3805)
  arc A259 (17.3064, 20.3973) -> (17.5422, 20.3805) centre (17.4358, 20.5498) ccw
  arc A260 (17.3064, 20.3973) -> (16.8243, 20.7968) centre (0, 0) ccw
  arc A261 (16.7639, 21.0253) -> (16.8243, 20.7968) centre (16.9501, 20.9523) ccw
  line L260 (16.7639, 21.0253) -> (17.1717, 22.0645)
  line L261 (17.4133, 22.8838) -> (17.1717, 22.0645)
  arc A262 (17.4133, 22.8838) -> (17.3037, 23.21) centre (17.1255, 22.9686) ccw
  line L262 (17.3037, 23.21) -> (17.0785, 23.3762)
  arc A263 (17.0785, 23.3762) -> (16.7345, 23.3848) centre (16.9004, 23.1348) ccw
  line L263 (16.7345, 23.3848) -> (16.0228, 22.9125)
  line L264 (16.0228, 22.9125) -> (15.15, 22.2164)
  arc A264 (14.9138, 22.2068) -> (15.15, 22.2164) centre (15.0253, 22.3728) ccw
  arc A265 (14.9138, 22.2068) -> (14.39, 22.5497) centre (0, 0) ccw
  arc A266 (14.3044, 22.7701) -> (14.39, 22.5497) centre (14.4976, 22.7183) ccw
  line L265 (14.3044, 22.7701) -> (14.5933, 23.8484)
  line L266 (14.5933, 23.8484) -> (14.7416, 24.6896)
  arc A267 (14.7416, 24.6896) -> (14.5962, 25.0015) centre (14.4462, 24.7417) ccw
  line L267 (14.5962, 25.0015) -> (14.3538, 25.1414)
  arc A268 (14.3538, 25.1414) -> (14.011, 25.1114) centre (14.2038, 24.8816) ccw
  line L268 (14.011, 25.1114) -> (13.3567, 24.5624)
  line L269 (13.3567, 24.5624) -> (12.5673, 23.773)
  arc A269 (12.3337, 23.737) -> (12.5673, 23.773) centre (12.4259, 23.9144) ccw
  arc A270 (12.3337, 23.737) -> (11.7747, 24.0191) centre (0, 0) ccw
  arc A271 (11.665, 24.2285) -> (11.7747, 24.0191) centre (11.8628, 24.1987) ccw
  line L270 (11.665, 24.2285) -> (11.8314, 25.3324)
  line L271 (11.8314, 25.3324) -> (11.8846, 26.1849)
  arc A272 (11.8846, 26.1849) -> (11.7051, 26.4785) centre (11.5852, 26.2035) ccw
  line L272 (11.7051, 26.4785) -> (11.4486, 26.5904)
  arc A273 (11.4486, 26.5904) -> (11.1113, 26.5222) centre (11.3286, 26.3155) ccw
  line L273 (11.1113, 26.5222) -> (10.5226, 25.9034)
  line L274 (10.5226, 25.9034) -> (9.8265, 25.0306)
  arc A274 (9.5984, 24.9686) -> (9.8265, 25.0306) centre (9.6702, 25.1553) ccw
  arc A275 (9.5984, 24.9686) -> (9.0114, 25.1864) centre (0, 0) ccw
  arc A276 (8.8789, 25.3822) -> (9.0114, 25.1864) centre (9.0788, 25.3748) ccw
  line L275 (8.8789, 25.3822) -> (8.9207, 26.4978)
  line L276 (8.9207, 26.4978) -> (8.8781, 27.3509)
  arc A277 (8.8781, 27.3509) -> (8.6669, 27.6226) centre (8.5785, 27.3359) ccw
  line L277 (8.3994, 27.7051) -> (8.6669, 27.6226)
  arc A278 (8.3994, 27.7051) -> (8.0719, 27.5995) centre (8.311, 27.4184) ccw
  line L278 (8.0719, 27.5995) -> (7.5562, 26.9187)
  line L279 (7.5562, 26.9187) -> (6.9622, 25.9735)
  arc A279 (6.7425, 25.8863) -> (6.9622, 25.9735) centre (6.7929, 26.0799) ccw
  circle A280 centre (5.2865, -10.0026) radius 2.0389
  circle A281 centre (-5.2865, 10.0026) radius 2.0389
  line L280 (-7.2999, -0.6404) -> (-10.1412, -1.2889)
  arc A282 (-10.1412, -1.2889) -> (-11.6123, -1.6247) centre (-10.0026, -5.2865) ccw
  line L281 (-11.6123, -1.6247) -> (-25.1128, -4.7061)
  arc A283 (-24.6909, 6.5697) -> (-25.1128, -4.7061) centre (0, 0) ccw
  line L282 (-24.6909, 6.5697) -> (-7.2316, 1.1842)
  arc A284 (-7.2316, 1.1842) -> (-7.2999, -0.6404) centre (0, 0) ccw
  line L283 (-24.6678, -6.656) -> (-13.8484, -4.1865)
  arc A285 (-13.8484, -4.1865) -> (-11.2601, -9.0837) centre (-10.0026, -5.2865) ccw
  line L284 (-11.2601, -9.0837) -> (-19.3953, -16.632)
  arc A286 (-24.6678, -6.656) -> (-19.3953, -16.632) centre (0, 0) ccw
  line L285 (-18.035, -18.0981) -> (-7.8838, -8.6793)
  arc A287 (-7.8838, -8.6793) -> (-6.7777, -7.653) centre (-10.0026, -5.2865) ccw
  line L286 (-6.7777, -7.653) -> (-4.6413, -5.6707)
  arc A288 (-4.6413, -5.6707) -> (-3.0953, -6.6421) centre (0, 0) ccw
  line L287 (-8.4808, -24.1014) -> (-3.0953, -6.6421)
  arc A289 (-18.035, -18.0981) -> (-8.4808, -24.1014) centre (0, 0) ccw
  line L288 (0.6404, -7.2999) -> (1.2889, -10.1412)
  arc A290 (1.2889, -10.1412) -> (1.6247, -11.6123) centre (5.2865, -10.0026) ccw
  line L289 (1.6247, -11.6123) -> (4.7061, -25.1128)
  arc A291 (-6.5697, -24.6909) -> (4.7061, -25.1128) centre (0, 0) ccw
  line L290 (-6.5697, -24.6909) -> (-1.1842, -7.2316)
  arc A292 (-1.1842, -7.2316) -> (0.6404, -7.2999) centre (0, 0) ccw
  line L291 (6.656, -24.6678) -> (4.1865, -13.8484)
  arc A293 (4.1865, -13.8484) -> (9.0837, -11.2601) centre (5.2865, -10.0026) ccw
  line L292 (9.0837, -11.2601) -> (16.632, -19.3953)
  arc A294 (6.656, -24.6678) -> (16.632, -19.3953) centre (0, 0) ccw
  line L293 (18.0981, -18.035) -> (8.6793, -7.8838)
  arc A295 (8.6793, -7.8838) -> (7.653, -6.7777) centre (5.2865, -10.0026) ccw
  line L294 (7.653, -6.7777) -> (5.6707, -4.6413)
  arc A296 (5.6707, -4.6413) -> (6.6421, -3.0953) centre (0, 0) ccw
  line L295 (24.1014, -8.4808) -> (6.6421, -3.0953)
  arc A297 (18.0981, -18.035) -> (24.1014, -8.4808) centre (0, 0) ccw
  line L296 (7.2999, 0.6404) -> (10.1412, 1.2889)
  arc A298 (10.1412, 1.2889) -> (11.6123, 1.6247) centre (10.0026, 5.2865) ccw
  line L297 (11.6123, 1.6247) -> (25.1128, 4.7061)
  arc A299 (24.6909, -6.5697) -> (25.1128, 4.7061) centre (0, 0) ccw
  line L298 (24.6909, -6.5697) -> (7.2316, -1.1842)
  arc A300 (7.2316, -1.1842) -> (7.2999, 0.6404) centre (0, 0) ccw
  line L299 (24.6678, 6.656) -> (13.8484, 4.1865)
  arc A301 (13.8484, 4.1865) -> (11.2601, 9.0837) centre (10.0026, 5.2865) ccw
  line L300 (11.2601, 9.0837) -> (19.3953, 16.632)
  arc A302 (24.6678, 6.656) -> (19.3953, 16.632) centre (0, 0) ccw
  line L301 (18.035, 18.0981) -> (7.8838, 8.6793)
  arc A303 (7.8838, 8.6793) -> (6.7777, 7.653) centre (10.0026, 5.2865) ccw
  line L302 (6.7777, 7.653) -> (4.6413, 5.6707)
  arc A304 (4.6413, 5.6707) -> (3.0953, 6.6421) centre (0, 0) ccw
  line L303 (8.4808, 24.1014) -> (3.0953, 6.6421)
  arc A305 (18.035, 18.0981) -> (8.4808, 24.1014) centre (0, 0) ccw
  line L304 (-0.6404, 7.2999) -> (-1.2889, 10.1412)
  arc A306 (-1.2889, 10.1412) -> (-1.6247, 11.6123) centre (-5.2865, 10.0026) ccw
  line L305 (-1.6247, 11.6123) -> (-4.7061, 25.1128)
  arc A307 (6.5697, 24.6909) -> (-4.7061, 25.1128) centre (0, 0) ccw
  line L306 (6.5697, 24.6909) -> (1.1842, 7.2316)
  arc A308 (1.1842, 7.2316) -> (-0.6404, 7.2999) centre (0, 0) ccw
  line L307 (-6.656, 24.6678) -> (-4.1865, 13.8484)
  arc A309 (-4.1865, 13.8484) -> (-9.0837, 11.2601) centre (-5.2865, 10.0026) ccw
  line L308 (-9.0837, 11.2601) -> (-16.632, 19.3953)
  arc A310 (-6.656, 24.6678) -> (-16.632, 19.3953) centre (0, 0) ccw
  line L309 (-18.0981, 18.035) -> (-8.6793, 7.8838)
  arc A311 (-8.6793, 7.8838) -> (-7.653, 6.7777) centre (-5.2865, 10.0026) ccw
  line L310 (-7.653, 6.7777) -> (-5.6707, 4.6413)
  arc A312 (-5.6707, 4.6413) -> (-6.6421, 3.0953) centre (0, 0) ccw
  line L311 (-24.1014, 8.4808) -> (-6.6421, 3.0953)
  arc A313 (-18.0981, 18.035) -> (-24.1014, 8.4808) centre (0, 0) ccw
  circle A314 centre (0, 0) radius 6
  circle A315 centre (10.0026, 5.2865) radius 2.0389
  circle A316 centre (-10.0026, -5.2865) radius 2.0389
  point P0 (0, 0)
  constraints: 624 end point, 624 point on circle, 317 centre point
extrude "Extrusion1" add sketch "Sketch1" along normal blind 7 contours A279 L279 L278 A278 L277 A277 L276 L275 A276 A275 A274 L274 L273 A273 L272 A272 L271 L270 A271 A270 A269 L269 L268 A268 L267 A267 L266 L265 A266 A265 A264 L264 L263 A263 L262 A262 L261 L260 A261 A260 A259 L259 L258 A258 L257 A257 L256 L255 A256 A255 A254 L254 L253 A253 L252 A252 L251 L250 A251 A250 A249 L249 L248 A248 L247 A247 L246 L245 A246 A245 A244 L244 L243 A243 L242 A242 L241 L240 A241 A240 A239 L239 L238 A238 L237 A237 L236 L235 A236 A235 A234 L234 L233 A233 L232 A232 L231 L230 A231 A230 A229 L229 L228 A228 L227 A227 L226 L225 A226 A225 A224 L224 L223 A223 L222 A222 L221 L220 A221 A220 A219 L219 L218 A218 L217 A217 L216 L215 A216 A215 A214 L214 L213 A213 L212 A212 L211 L210 A211 A210 A209 L209 L208 A208 L207 A207 L206 L205 A206 A205 A204 L204 L203 A203 L202 A202 L201 L200 A201 A200 A199 L199 L198 A198 L197 A197 L196 L195 A196 A195 A194 L194 L193 A193 L192 A192 L191 L190 A191 A190 A189 L189 L188 A188 L187 A187 L186 L185 A186 A185 A184 L184 L183 A183 L182 A182 L181 L180 A181 A180 A179 L179 L178 A178 L177 A177 L176 L175 A176 A175 A174 L174 L173 A173 L172 A172 L171 L170 A171 A170 A169 L169 L168 A168 L167 A167 L166 L165 A166 A165 A164 L164 L163 A163 L162 A162 L161 L160 A161 A160 A159 L159 L158 A158 L157 A157 L156 L155 A156 A155 A154 L154 L153 A153 L152 A152 L151 L150 A151 A150 A149 L149 L148 A148 L147 A147 L146 L145 A146 A145 A144 L144 L143 A143 L142 A142 L141 L140 A141 A140 A139 L139 L138 A138 L137 A137 L136 L135 A136 A135 A134 L134 L133 A133 L132 A132 L131 L130 A131 A130 A129 L129 L128 A128 L127 A127 L126 L125 A126 A125 A124 L124 L123 A123 L122 A122 L121 L120 A121 A120 A119 L119 L118 A118 L117 A117 L116 L115 A116 A115 A114 L114 L113 A113 L112 A112 L111 L110 A111 A110 A109 L109 L108 A108 L107 A107 L106 L105 A106 A105 A104 L104 L103 A103 L102 A102 L101 L100 A101 A100 A99 L99 L98 A98 L97 A97 L96 L95 A96 A95 A94 L94 L93 A93 L92 A92 L91 L90 A91 A90 A89 L89 L88 A88 L87 A87 L86 L85 A86 A85 A84 L84 L83 A83 L82 A82 L81 L80 A81 A80 A79 L79 L78 A78 L77 A77 L76 L75 A76 A75 A74 L74 L73 A73 L72 A72 L71 L70 A71 A70 A69 L69 L68 A68 L67 A67 L66 L65 A66 A65 A64 L64 L63 A63 L62 A62 L61 L60 A61 A60 A59 L59 L58 A58 L57 A57 L56 L55 A56 A55 A54 L54 L53 A53 L52 A52 L51 L50 A51 A50 A49 L49 L48 A48 L47 A47 L46 L45 A46 A45 A44 L44 L43 A43 L42 A42 L41 L40 A41 A40 A39 L39 L38 A38 L37 A37 L36 L35 A36 A35 A34 L34 L33 A33 L32 A32 L31 L30 A31 A30 A29 L29 L28 A28 L27 A27 L26 L25 A26 A25 A24 L24 L23 A23 L22 A22 L21 L20 A21 A20 A19 L19 L18 A18 L17 A17 L16 L15 A16 A15 A14 L14 L13 A13 L12 A12 L11 L10 A11 A10 A9 L9 L8 A8 L7 A7 L6 L5 A6 A5 A4 L4 L3 A3 L2 A2 L1 L0 A1 A0 | L280 A282 L281 A283 L282 A284 | L283 A285 L284 A286 | L285 A287 L286 A288 L287 A289 | L288 A290 L289 A291 L290 A292 | L291 A293 L292 A294 | L293 A295 L294 A296 L295 A297 | L296 A298 L297 A299 L298 A300 | L299 A301 L300 A302 | L301 A303 L302 A304 L303 A305 | L304 A306 L305 A307 L306 A308 | L307 A309 L308 A310 | L309 A311 L310 A312 L311 A313
extrude "Extrusion2" cut sketch "Sketch1" along normal blind 1.5 contours L280 A282 L281 A283 L282 A284 | L283 A285 L284 A286 | L285 A287 L286 A288 L287 A289 | L288 A290 L289 A291 L290 A292 | L291 A293 L292 A294 | L293 A295 L294 A296 L295 A297 | L296 A298 L297 A299 L298 A300 | L299 A301 L300 A302 | L301 A303 L302 A304 L303 A305 | L304 A306 L305 A307 L306 A308 | L307 A309 L308 A310 | L309 A311 L310 A312 L311 A313
ref_plane "Work Plane1" through (0, 3.5, 0) normal (0, -1, 0) x (1, 0, 0)
mirror "Mirror1" about plane through (0, 3.5, 0) normal (0, -1, 0) of "Extrusion2"
body "Solid1"
